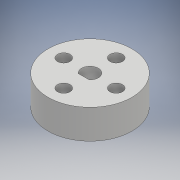
# Autodesk Inventor part: sleeve for kick
Saved by Autodesk Inventor 2018 (Build 220112000, 112)
## iProperties
Created: 2019-11-13
Part Number: sleeve for kick
Material: Типовые
Document SubType Name: Modeling
Designer: cosko
Density: 1 g/cm^3
Appearance: По умолчанию
Author: cosko
Autodesk Inventor part; units mm, degrees
ref_plane "YZ Plane" through (0, 0, 0) normal (1, 0, 0) x (0, 1, 0)
ref_plane "XZ Plane" through (0, 0, 0) normal (0, 1, 0) x (-1, 0, 0)
ref_plane "XY Plane" through (0, 0, 0) normal (0, 0, 1) x (1, 0, 0)
sketch "Эскиз1" plane through (0, 0, 0) normal (0, 0, 1) x (1, 0, 0)
  circle A0 centre (0, 0) radius 10
  line L0 (0, 0) -> (-6.25, 0) construction
  line L1 (0, 0) -> (6.25, 0) construction
  circle A1 centre (-6.25, 0) radius 1.5
  circle A2 centre (6.25, 0) radius 1.5
  circle A3 centre (0, -6.25) radius 1.5
  circle A4 centre (0, 6.25) radius 1.5
  line L2 (0, 0) -> (0, -6.25) construction
  line L3 (0, 0) -> (0, 6.25) construction
  arc A5 (1.3229, -1.5) -> (-1.3229, -1.5) centre (0, 0) ccw
  line L4 (0, 0) -> (0, -1.5) construction
  line L5 (1.3229, -1.5) -> (-1.3229, -1.5)
  dimension "d0" = 20
  dimension "d1" = 6.25
  dimension "d2" = 6.25
  dimension "d3" = 3
  dimension "d4" = 3
  dimension "d7" = 90
  dimension "d9" = 4
  dimension "d10" = 1.5
  constraints: 12 end point, 6 centre point, 6 coincident, 3 horizontal, 2 point on circle, 1 point on line, 10 other
  measures "d0" diameter of A0
  measures "d1" distance of L0.start L0.end
  measures "d2" distance of L0.start L1.end
  measures "d3" diameter of A1
  measures "d4" diameter of A2
  measures "d9" diameter of A5
  measures "d10" distance of L4.start L4.end
extrude "Выдавливание1" add sketch "Эскиз1" along normal blind 7
